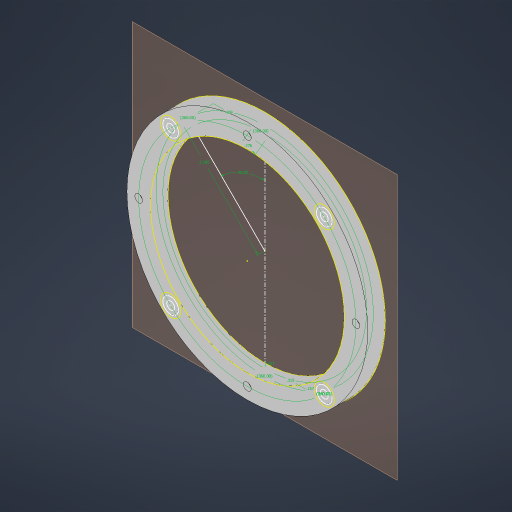
# Autodesk Inventor part: TopSpacer
Saved by Autodesk Inventor 2024 (Build 280153000, 153)
## iProperties
Created: 2023-10-21
Part Number: TopSpacer
Material: Generic
Document SubType Name: Modeling
Designer: range
Density: 1 g/cm^3
Appearance: Default
Author: range
Autodesk Inventor part; units mm, degrees
ref_plane "YZ Plane" through (0, 0, 0) normal (1, 0, 0) x (0, 1, 0)
ref_plane "XZ Plane" through (0, 0, 0) normal (0, 1, 0) x (-1, 0, 0)
ref_plane "XY Plane" through (0, 0, 0) normal (0, 0, 1) x (1, 0, 0)
ref_plane "Work Plane1" through (0, 0, 0) normal (0, 0, 1) x (1, 0, 0)
sketch "Sketch1" plane through (0, 0, 0) normal (0, 0, 1) x (1, 0, 0)
  circle A0 centre (0, -55.5) radius 5.1943 projected
  circle A1 centre (-55.5, 0) radius 5.1943 projected
  circle A2 centre (0, 55.5) radius 5.1943 projected
  circle A3 centre (55.5, 0) radius 5.1943 projected
  circle A4 centre (0, 0) radius 61.5 projected
  circle A5 centre (0, 0) radius 49.5 projected
  line L0 (-2.0207, 52) -> (-4.0415, 55.5)
  line L1 (-4.0415, 55.5) -> (-2.0207, 59)
  line L2 (-2.0207, 59) -> (2.0207, 59)
  line L3 (2.0207, 59) -> (4.0415, 55.5)
  line L4 (4.0415, 55.5) -> (2.0207, 52)
  line L5 (2.0207, 52) -> (-2.0207, 52)
  line L6 (0, 55.5) -> (0, 52) construction
  line L7 (-52, -2.0207) -> (-55.5, -4.0415)
  line L8 (-55.5, -4.0415) -> (-59, -2.0207)
  line L9 (-59, -2.0207) -> (-59, 2.0207)
  line L10 (-59, 2.0207) -> (-55.5, 4.0415)
  line L11 (-55.5, 4.0415) -> (-52, 2.0207)
  line L12 (-52, 2.0207) -> (-52, -2.0207)
  line L13 (2.0207, -52) -> (4.0415, -55.5)
  line L14 (4.0415, -55.5) -> (2.0207, -59)
  line L15 (2.0207, -59) -> (-2.0207, -59)
  line L16 (-2.0207, -59) -> (-4.0415, -55.5)
  line L17 (-4.0415, -55.5) -> (-2.0207, -52)
  line L18 (-2.0207, -52) -> (2.0207, -52)
  line L19 (52, 2.0207) -> (55.5, 4.0415)
  line L20 (55.5, 4.0415) -> (59, 2.0207)
  line L21 (59, 2.0207) -> (59, -2.0207)
  line L22 (59, -2.0207) -> (55.5, -4.0415)
  line L23 (55.5, -4.0415) -> (52, -2.0207)
  line L24 (52, -2.0207) -> (52, 2.0207)
  circle A6 centre (0, 55.5) radius 5.1943
  circle A7 centre (-39.2444, 39.2444) radius 5.1943
  line L25 (-39.2444, 39.2444) -> (0, 0)
  line L26 (0, 55.5) -> (0, -55.5)
  circle A8 centre (-39.2444, -39.2444) radius 5.1943
  circle A9 centre (39.2444, -39.2444) radius 5.1943
  circle A10 centre (39.2444, 39.2444) radius 5.1943
  circle A11 centre (0, -55.5) radius 2
  circle A12 centre (55.5, 0) radius 2
  circle A13 centre (0, 55.5) radius 2
  circle A14 centre (-55.5, 0) radius 2
  point P0 (-52, 0)
  point P1 (0, -52)
  point P2 (52, 0)
  dimension "d2" = 7
  dimension "d5" = 360
  dimension "d11" = 45
  dimension "d12" = 10.3886
  dimension "d13" = 55.5
  dimension "d16" = 360
  dimension "d32" = 4
  dimension "d35" = 360
  constraints: 54 end point, 9 centre point, 3 coincident, 2 vertical, 1 concentric, 1 midpoint, 84 other
  measures "d2" distance between parallel lines of L4 L1
  measures "d11" angle of L25 L26
  measures "d12" diameter of A7
  measures "d13" distance of L25.start L25.end
  measures "d32" diameter of A11
extrude "Extrusion1" add sketch "Sketch1" along normal blind 8.89 contours A11 | L18 L13 L14 L15 L16 L17 | A0 | A7 | A13 | L5 L0 L1 L2 L3 L4 | A2 | A1 | A3 | A4 | L7 L8 L9 L10 L11 L12 | L19 L20 L21 L22 L23 L24 | A8 | A9 | A10 | A12 | A14
extrude "Extrusion2" cut sketch "Sketch1" along normal blind 6.35 contours A11 | L18 L13 L14 L15 L16 L17 | A13 | L5 L0 L1 L2 L3 L4 | L7 L8 L9 L10 L11 L12 | L19 L20 L21 L22 L23 L24 | A12 | A14
sketch "Sketch2" plane through (0, 0, 8.89) normal (0, 0, 1) x (1, 0, 0)
  circle A0 centre (39.2444, 39.2444) radius 5.1943 projected
  circle A1 centre (39.2444, -39.2444) radius 5.1943 projected
  circle A2 centre (-39.2444, -39.2444) radius 5.1943 projected
  circle A3 centre (-39.2444, 39.2444) radius 5.1943 projected
  circle A4 centre (39.2444, -39.2444) radius 4
  circle A5 centre (0, 0) radius 49.5 projected
  circle A6 centre (39.2444, 39.2444) radius 4
  circle A7 centre (-39.2444, 39.2444) radius 4
  circle A8 centre (-39.2444, -39.2444) radius 4
  circle A9 centre (39.2444, -39.2444) radius 2
  circle A10 centre (39.2444, 39.2444) radius 2
  circle A11 centre (-39.2444, 39.2444) radius 2
  circle A12 centre (-39.2444, -39.2444) radius 2
  dimension "d18" = 8
  dimension "d21" = 360
  dimension "d25" = 4
  dimension "d28" = 360
  constraints: 8 centre point, 2 coincident, 18 other
  measures "d18" diameter of A4
  measures "d25" diameter of A9
extrude "Extrusion3" cut sketch "Sketch2" against normal blind 6.35 contours A4 | A6 | A7 | A8 | A9 | A10 | A11 | A12
extrude "Extrusion4" cut sketch "Sketch2" against normal blind 15.875 contours A9 | A10 | A11 | A12
extrude "Extrusion5" cut sketch "Sketch1" along normal through all contours A11 | A13 | A12 | A14
body "Solid1"
